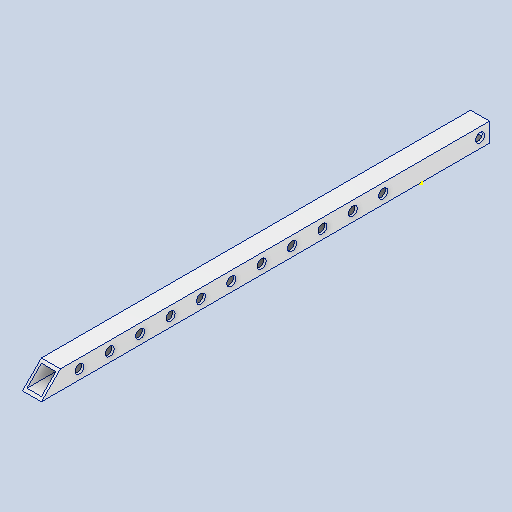
# Autodesk Inventor part: P701
Saved by Autodesk Inventor 2023 (Build 270158000, 158)
## iProperties
Created: 2022-08-23
Part Number: P701
Material: Aluminum 6061
Document SubType Name: Modeling
Designer: D.C. Eksteen
Density: 2.7 g/cm^3
Appearance: Aluminum - Flat
Mass: 238.696 g
Surface Area: 901.563 cm^2
Volume: 88.406 cm^3
Author: D.C. Eksteen
Title: FRONT FRAME LEFT BRACKET
Autodesk Inventor part; units mm, degrees
ref_plane "YZ Plane" through (0, 0, 0) normal (1, 0, 0) x (0, 1, 0)
ref_plane "XZ Plane" through (0, 0, 0) normal (0, 1, 0) x (-1, 0, 0)
ref_plane "XY Plane" through (0, 0, 0) normal (0, 0, 1) x (1, 0, 0)
sketch "Sketch1" plane through (0, 0, 0) normal (0, 0, 1) x (1, 0, 0)
  line L0 (0, 0) -> (25, 0)
  line L1 (25, 0) -> (25, 25)
  line L2 (25, 25) -> (0, 25)
  line L3 (0, 25) -> (0, 0)
  line L4 (3, 3) -> (22, 3)
  line L5 (22, 3) -> (22, 22)
  line L6 (22, 22) -> (3, 22)
  line L7 (3, 22) -> (3, 3)
  dimension "d0" = 25
  dimension "d1" = 25
  dimension "d2" = 3
  constraints: 16 end point, 4 parallel, 2 perpendicular, 1 horizontal, 3 other
  measures "d0" distance of L2.end L1.end
  measures "d1" distance of L1.end L0.end
  measures "d2" distance between parallel lines of L3 L7
extrude "Extrusion1" add sketch "Sketch1" along normal blind 500
sketch "Sketch3" plane through (25, 0, 0) normal (1, 0, 0) x (0, 0, -1)
  line L0 (0, 0) -> (0, 25) projected
  line L1 (0, 25) -> (-500, 25) projected
  line L2 (-500, 0) -> (-500, 25) projected
  line L3 (0, 0) -> (-500, 0) projected
  point P0 (0, 0)
  point P1 (-450, 12.5)
  point P2 (-50, 12.5)
  point P3 (-410, 12.5)
  point P4 (-370, 12.5)
  point P5 (-330, 12.5)
  point P6 (-290, 12.5)
  point P7 (-250, 12.5)
  point P8 (-210, 12.5)
  point P9 (-170, 12.5)
  point P10 (-130, 12.5)
  point P11 (-90, 12.5)
  dimension "d16" = 12.5
  dimension "d17" = 50
  dimension "d18" = 50
  dimension "d19" = 12.5
  dimension "d22" = 40
  constraints: 1 horizontal, 9 other
  measures "d16" distance from line of L3 point (-450, 12.5)
  measures "d17" distance from line of L2 point (-450, 12.5)
  measures "d18" distance from line of L0 point (-50, 12.5)
  measures "d19" distance from line of L3 point (-50, 12.5)
  measures "d22" distance of point (-450, 12.5) point (-410, 12.5)
hole "Hole2" at (25, 12.5, 450) at (25, 12.5, 50) at (25, 12.5, 410) at (25, 12.5, 370) at (25, 12.5, 330) at (25, 12.5, 290) at (25, 12.5, 250) at (25, 12.5, 210) at (25, 12.5, 170) at (25, 12.5, 130) at (25, 12.5, 90) direction (-1, 0, 0) diameter 12 depth 8 tip angle 118
sketch "Sketch4" plane through (3, 3, 0) normal (1, 0, 0) x (0, 0, -1)
  circle A0 centre (-130, 9.5) radius 6 projected
  circle A1 centre (-210, 9.5) radius 6 projected
  circle A2 centre (-290, 9.5) radius 6 projected
  circle A3 centre (-370, 9.5) radius 6 projected
  circle A4 centre (-50, 9.5) radius 6 projected
  circle A5 centre (-450, 9.5) radius 6 projected
  circle A6 centre (-410, 9.5) radius 6 projected
  circle A7 centre (-330, 9.5) radius 6 projected
  circle A8 centre (-250, 9.5) radius 6 projected
  circle A9 centre (-170, 9.5) radius 6 projected
  circle A10 centre (-90, 9.5) radius 6 projected
  line L0 (0, -3) -> (0, 22) projected
  line L1 (0, 22) -> (-500, 22) projected
  line L2 (-500, -3) -> (-500, 22) projected
  line L3 (0, -3) -> (-500, -3) projected
  arc A11 (0, -3) -> (0, -3) centre (-50, 9.5) ccw projected
  circle A12 centre (-210, 9.5) radius 6 projected
  circle A13 centre (-250, 9.5) radius 6 projected
  circle A14 centre (-370, 9.5) radius 6 projected
  circle A15 centre (-410, 9.5) radius 6 projected
  constraints: 11 coincident, 1 other
hole "Hole3" at (3, 12.5, 50) at (3, 12.5, 90) at (3, 12.5, 130) at (3, 12.5, 170) at (3, 12.5, 210) at (3, 12.5, 250) at (3, 12.5, 290) at (3, 12.5, 330) at (3, 12.5, 370) at (3, 12.5, 410) at (3, 12.5, 450) direction (-1, 0, 0) diameter 7 depth 8 tip angle 118
sketch "Sketch6" plane through (0, 0, 0) normal (0, 0, -1) x (-1, 0, 0)
  line L0 (-25, 0) -> (-25, 25) projected
  line L1 (0, 0) -> (-25, 0) projected
  line L2 (0, 25) -> (0, 0) projected
  line L3 (-25, 25) -> (0, 25) projected
  line L4 (-3, 3) -> (-3, 22) projected
  line L5 (-22, 3) -> (-3, 3) projected
  line L6 (-22, 22) -> (-22, 3) projected
  line L7 (-3, 22) -> (-22, 22) projected
extrude "Extrusion3" add sketch "Sketch6" along normal blind 90
sketch "Sketch7" plane through (0, 0, 500) normal (-1, 0, 0) x (0, 0, 1)
  circle A0 centre (-90, 12.5) radius 3.5 projected
  circle A1 centre (-170, 12.5) radius 3.5 projected
  circle A2 centre (-250, 12.5) radius 3.5 projected
  circle A3 centre (-330, 12.5) radius 3.5 projected
  circle A4 centre (-410, 12.5) radius 3.5 projected
  circle A5 centre (-450, 12.5) radius 3.5 projected
  circle A6 centre (-370, 12.5) radius 3.5 projected
  circle A7 centre (-290, 12.5) radius 3.5 projected
  circle A8 centre (-210, 12.5) radius 3.5 projected
  circle A9 centre (-130, 12.5) radius 3.5 projected
  circle A10 centre (-50, 12.5) radius 3.5 projected
  line L0 (-590, 0) -> (0, 0) projected
  line L1 (0, 25) -> (0, 0) projected
  line L2 (-590, 25) -> (0, 25) projected
  line L3 (-590, 0) -> (-590, 25) projected
  point P0 (-500, 0)
  point P1 (-577.5, 12.5)
  dimension "d47" = 12.5
  dimension "d48" = 12.5
  measures "d47" distance from line of L2 point (-577.5, 12.5)
  measures "d48" distance from line of L3 point (-577.5, 12.5)
hole "Hole4" at (0, 12.5, -77.5) direction (1, 0, 0) diameter 12 end through all
sketch "Sketch8" plane through (25, 0, 500) normal (1, 0, 0) x (0, 0, -1)
  point P0 (500, 0)
sketch "Sketch9" plane through (0, 0, 500) normal (-1, 0, 0) x (0, 0, 1)
  circle A0 centre (-577.5, 12.5) radius 6 projected
  circle A1 centre (-90, 12.5) radius 3.5 projected
  circle A2 centre (-170, 12.5) radius 3.5 projected
  circle A3 centre (-250, 12.5) radius 3.5 projected
  circle A4 centre (-330, 12.5) radius 3.5 projected
  circle A5 centre (-410, 12.5) radius 3.5 projected
  circle A6 centre (-450, 12.5) radius 3.5 projected
  circle A7 centre (-370, 12.5) radius 3.5 projected
  circle A8 centre (-290, 12.5) radius 3.5 projected
  circle A9 centre (-210, 12.5) radius 3.5 projected
  circle A10 centre (-130, 12.5) radius 3.5 projected
  circle A11 centre (-50, 12.5) radius 3.5 projected
  line L0 (-590, 0) -> (0, 0) projected
  line L1 (0, 25) -> (0, 0) projected
  line L2 (-590, 25) -> (0, 25) projected
  line L3 (-590, 0) -> (-590, 25) projected
  line L4 (0, 0) -> (0, 25) projected
  line L5 (0, 0) -> (-25, 25)
  line L6 (-590, 25) -> (0, 25) projected
  point P0 (-500, 0)
  dimension "d56" = 45
  constraints: 2 end point, 1 point on line
  measures "d56" angle of L1 L5
extrude "Extrusion4" cut sketch "Sketch9" against normal blind 109.75 contours L5 L2 L1
body "Solid1"
